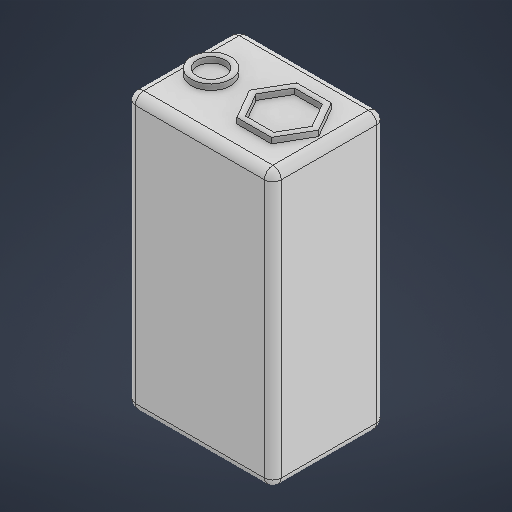
# Autodesk Inventor part: bateria IC
Saved by Autodesk Inventor 2026.2 (Build 302298010, 298A)
## iProperties
Created: 2026-03-28
Part Number: bateria IC
Material: Genérico
Document SubType Name: Modeling
Designer: Lucas David
Density: 1 g/cm^3
Appearance: Padrão
Author: Lucas David
Autodesk Inventor part; units mm, degrees
ref_plane "YZ Plane" through (0, 0, 0) normal (1, 0, 0) x (0, 1, 0)
ref_plane "XZ Plane" through (0, 0, 0) normal (0, 1, 0) x (-1, 0, 0)
ref_plane "XY Plane" through (0, 0, 0) normal (0, 0, 1) x (1, 0, 0)
sketch "Esboço1" plane through (0, 0, 0) normal (0, 0, 1) x (1, 0, 0)
  line L0 (-13, -24.5) -> (13, -24.5)
  line L1 (13, -24.5) -> (13, 24.5)
  line L2 (13, 24.5) -> (-13, 24.5)
  line L3 (-13, 24.5) -> (-13, -24.5)
  line L4 (-13, -24.5) -> (13, 24.5) construction
  line L5 (13, -24.5) -> (-13, 24.5) construction
  point P0 (0, 0)
  dimension "d0" = 49
  dimension "d1" = 26
  constraints: 12 end point, 2 midpoint, 2 parallel, 1 horizontal, 1 perpendicular
  measures "d0" distance between parallel lines of L0 L2
  measures "d1" distance between parallel lines of L1 L3
extrude "Extrusão1" add sketch "Esboço1" along normal blind 20
sketch "Esboço2" plane through (-13, 24.5, 0) normal (0, 1, 0) x (1, 0, 0)
  circle A0 centre (5, -10) radius 2.5
  line L0 (26, 0) -> (0, 0) projected
  line L1 (0, 0) -> (0, -20) projected
  line L2 (26, -20) -> (0, -20) projected
  line L3 (26, 0) -> (26, -20) projected
  line L4 (20.5, -14.3301) -> (15.5, -14.3301)
  line L5 (15.5, -14.3301) -> (13, -10)
  line L6 (13, -10) -> (15.5, -5.6699)
  line L7 (15.5, -5.6699) -> (20.5, -5.6699)
  line L8 (20.5, -5.6699) -> (23, -10)
  line L9 (23, -10) -> (20.5, -14.3301)
  circle A1 centre (5, -10) radius 3.5
  line L10 (14.9226, -4.6699) -> (11.8453, -10)
  line L11 (11.8453, -10) -> (14.9226, -15.3301)
  line L12 (14.9226, -15.3301) -> (21.0774, -15.3301)
  line L13 (21.0774, -15.3301) -> (24.1547, -10)
  line L14 (24.1547, -10) -> (21.0774, -4.6699)
  line L15 (21.0774, -4.6699) -> (14.9226, -4.6699)
  point P0 (13, 0)
  point P1 (18, -10)
  dimension "d5" = 5
  dimension "d7" = 5
  dimension "d8" = 5
  dimension "d9" = 13
  dimension "d10" = 10
  dimension "d11" = 10
  dimension "d12" = 5
  dimension "d13" = 1
  dimension "d14" = 1
  constraints: 24 end point, 2 centre point, 18 other
  measures "d5" diameter of A0
  measures "d7" distance of L7.end L8.end
  measures "d8" distance of L6.end L7.end
  measures "d9" distance of A0.centre point (18, -10)
  measures "d10" distance from line of L2 A0.centre
  measures "d11" distance from line of L2 point (18, -10)
  measures "d12" distance from line of L1 A0.centre
  measures "d13" radial gap between concentric circles of A0 A1
  measures "d14" distance between parallel lines of L6 L10
extrude "Extrusão2" add sketch "Esboço2" along normal blind 1 contours A0 | L4 L5 L6 L7 L8 L9 | A1 | L15 L14 L13 L12 L11 L10
extrude "Extrusão3" cut sketch "Esboço2" against normal blind 1 from surface at 1 contours A0 | L4 L5 L6 L7 L8 L9
fillet "Arredondamento1" radius 1.5 12 edges at (-13, 0, 20) (13, 0, 20) (0, 24.5, 20) (13, 24.5, 10) (-13, 24.5, 10) (0, 24.5, 0) (-13, 0, 0) (-13, -24.5, 10) (0, -24.5, 20) (0, -24.5, 0) (13, -24.5, 10) (13, 0, 0)
